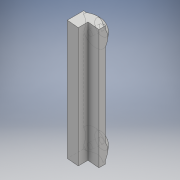
# Autodesk Inventor part: hbridge_module_holder
Saved by Autodesk Inventor 2018 (Build 220112000, 112)
## iProperties
Created: 2018-01-05
Part Number: hbridge_module_holder
Material: Generic
Document SubType Name: Modeling
Designer: erwin
Density: 1 g/cm^3
Appearance: Default
Author: erwin
Autodesk Inventor part; units mm, degrees
ref_plane "YZ Plane" through (0, 0, 0) normal (1, 0, 0) x (0, 1, 0)
ref_plane "XZ Plane" through (0, 0, 0) normal (0, 1, 0) x (-1, 0, 0)
ref_plane "XY Plane" through (0, 0, 0) normal (0, 0, 1) x (1, 0, 0)
sketch "Sketch1" plane through (0, 0, 0) normal (0, 1, 0) x (-1, 0, 0)
  line L0 (0, 0) -> (11, 0)
  line L1 (11, 0) -> (11, -55)
  line L2 (11, -55) -> (0, -55)
  line L3 (0, -55) -> (0, 0)
  dimension "d0" = 11
  dimension "d1" = 55
  constraints: 8 end point, 2 parallel, 1 horizontal, 1 perpendicular
  measures "d0" distance of L1.end L2.end
  measures "d1" distance of L0.end L1.end
extrude "Extrusion1" add sketch "Sketch1" along normal blind 4
sketch "Sketch2" plane through (-11, 0, 0) normal (0, 0, 1) x (1, 0, 0)
  line L0 (0, 4) -> (11, 4) projected
  line L1 (0, 4) -> (11, 3.0376)
  line L2 (11, 4) -> (16.9864, 4) construction
  line L3 (11, 0) -> (0, 0) projected
  line L4 (11, 3.0376) -> (11, 4)
  line L5 (0, 4) -> (11, 4) projected
  line L6 (0, 0) -> (0, 4) projected
  dimension "d4" = 5
  constraints: 6 end point, 1 horizontal, 1 point on line
  measures "d4" angle of L1 L2
extrude "Extrusion2" cut sketch "Sketch2" against normal through all
sketch "Sketch3" plane through (-11, 4, 0) normal (0.0871557, 0.9961947, 0) x (0.9961947, -0.0871557, 0)
  line L0 (0, 55) -> (11.042, 55) projected
  line L1 (11.042, 0) -> (0, 0) projected
  line L2 (0, 55) -> (0, 0) projected
  line L3 (11.042, 55) -> (11.042, 0) projected
  circle A0 centre (5.5, 50) radius 3.5
  point P0 (11.3068, 0)
  point P1 (5.5, 5)
  dimension "d7" = 45
  dimension "d9" = 5
  dimension "d11" = 5
  dimension "d12" = 5.5
  dimension "d13" = 5.542
  dimension "d14" = 5.5
  dimension "d15" = 7
  constraints: 1 centre point, 1 coincident
  measures "d7" distance of point (5.5, 5) point (5.5, 50)
  measures "d9" distance from line of L1 point (5.5, 5)
  measures "d11" distance from line of point (5.5, 50) L0
  measures "d12" distance from line of L2 point (5.5, 50)
  measures "d13" distance from line of L3 point (5.5, 50)
  measures "d14" distance from line of L2 point (5.5, 5)
  measures "d15" diameter of A0
extrude "Extrusion3" add sketch "Sketch3" along normal blind 3 contours A0
hole "Hole1" at (-5.2595, 6.5092, -50) direction (-0.0871557, -0.9961947, 0) diameter 2.5 depth 5
chamfer "Chamfer1" distance 3 angle 45 1 edges at (-9.0076, 3.8257, -50)
pattern_linear "Rectangular Pattern1" count 2 spacing 45 along (0, 0, 1) of "Extrusion3", "Chamfer1", "Hole1"
sketch "Sketch4" plane through (0, 0, 0) normal (0, -1, 0) x (1, 0, 0)
  line L0 (0, 0) -> (-11, 0) projected
  line L1 (-11, -55) -> (0, -55) projected
  line L2 (-11, 0) -> (-5.5, 0)
  line L3 (-5.5, 0) -> (-5.5, -55)
  line L4 (-5.5, -55) -> (-11, -55)
  line L5 (-11, -55) -> (-11, 0)
  constraints: 8 end point, 2 parallel, 1 horizontal, 1 midpoint, 1 perpendicular
extrude "Extrusion4" add sketch "Sketch4" along normal blind 4
sketch "Sketch5" plane through (0, 0, -55) normal (0, 0, -1) x (-1, 0, 0)
  line L0 (0, 0) -> (5.5, 0.4812)
  line L1 (0, 0) -> (19.5242, 0) construction
  line L2 (5.5, 0) -> (5.5, -4) projected
  line L3 (5.5, -4) -> (11.767, -3.4517)
  line L4 (5.5, 0.4812) -> (5.5, -4)
  line L5 (11.767, -3.4517) -> (11.767, -4.8815)
  line L6 (11.767, -4.8815) -> (1.8256, -4.7702)
  line L7 (1.8256, -4.7702) -> (0, 0)
  dimension "d36" = 5
  constraints: 14 end point, 1 collinear, 1 horizontal, 1 vertical
  measures "d36" angle of L1 L0
extrude "Extrusion5" cut sketch "Sketch5" against normal through all
equation "\"d11\" = d9"
equation "\"d14\" = d12"
body "Solid1"
